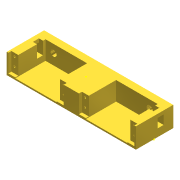
# Autodesk Inventor part: Part4
Saved by Autodesk Inventor 2022 (Build 260153000, 153)
## iProperties
Created: 2021-06-22
Part Number: Part4
Material: Generic
Document SubType Name: Modeling
Designer: Prajwal Patil
Density: 1 g/cm^3
Appearance: Diamond Plate
Author: Prajwal Patil
Autodesk Inventor part; units mm, degrees
ref_plane "YZ Plane" through (0, 0, 0) normal (1, 0, 0) x (0, 1, 0)
ref_plane "XZ Plane" through (0, 0, 0) normal (0, 1, 0) x (-1, 0, 0)
ref_plane "XY Plane" through (0, 0, 0) normal (0, 0, 1) x (1, 0, 0)
sketch "Sketch2" plane through (0, 0, 0) normal (0, 1, 0) x (-1, 0, 0)
  line L0 (77.2994, 22.4824) -> (-85.2606, 22.4824)
  line L1 (-85.2606, 22.4824) -> (-85.2606, -24.5076)
  line L2 (-85.2606, -24.5076) -> (77.2994, -24.5076)
  line L3 (77.2994, -24.5076) -> (77.2994, 22.4824)
  point P0 (0, 0)
  dimension "d0" = 162.56
  dimension "d1" = 46.99
  constraints: 8 end point, 2 parallel, 1 horizontal, 1 perpendicular
  measures "d0" distance of L2.end L1.end
  measures "d1" distance of L1.end L0.end
extrude "Extrusion1" add sketch "Sketch2" along normal blind 25.4
sketch "Sketch3" plane through (0, 25.4, 0) normal (0, 1, 0) x (1, 0, 0)
  point P0 (0, 0)
sketch "Sketch4" plane through (0, 25.4, 0) normal (0, 1, 0) x (1, 0, 0)
  line L0 (85.2606, -22.4824) -> (85.2606, 24.5076) projected
  line L1 (74.5926, -22.4824) -> (74.5926, 15.6176)
  line L2 (74.5926, 15.6176) -> (22.2686, 15.6176)
  line L3 (22.2686, 15.6176) -> (22.2686, -22.4824)
  line L4 (-14.3074, -22.4824) -> (-14.3074, 15.6176)
  line L5 (-14.3074, 15.6176) -> (-66.6314, 15.6176)
  line L6 (-66.6314, 15.6176) -> (-66.6314, -22.4824)
  line L7 (-66.6314, -22.4824) -> (-14.3074, -22.4824)
  line L8 (22.2686, -22.4824) -> (74.5926, -22.4824)
  point P0 (0, 0)
  dimension "d4" = 10.668
  dimension "d5" = 38.1
  dimension "d6" = 52.324
  dimension "d7" = 36.576
  dimension "d8" = 52.324
  constraints: 16 end point, 3 perpendicular, 1 collinear
  measures "d4" distance of L0.start L1.start
  measures "d5" distance of L1.start L1.end
  measures "d6" distance of L1.end L2.end
  measures "d7" distance of L3.end L4.start
  measures "d8" distance of L4.end L5.end
extrude "Extrusion2" cut sketch "Sketch4" against normal blind 23.495
sketch "Sketch5" plane through (0, 25.4, 0) normal (0, 1, 0) x (1, 0, 0)
  line L0 (74.5926, -22.4824) -> (22.2686, -22.4824) projected
  line L1 (22.2686, -22.4824) -> (13.5564, -22.4824)
  line L2 (13.5564, -22.4824) -> (13.5564, -18.6724)
  line L3 (13.5564, -18.6724) -> (22.2686, -18.6724)
  line L4 (22.2686, -18.6724) -> (22.2686, -22.4824)
  line L5 (-14.3074, -22.4824) -> (22.2686, -22.4824) projected
  line L6 (-14.3074, -22.4824) -> (-5.5952, -22.4824)
  line L7 (-5.5952, -22.4824) -> (-5.5952, -18.6724)
  line L8 (-5.5952, -18.6724) -> (-14.3074, -18.6724)
  line L9 (-14.3074, -18.6724) -> (-14.3074, -22.4824)
  line L10 (74.5926, -22.4824) -> (85.2606, -22.4824) projected
  line L11 (74.5926, -22.4824) -> (83.3048, -22.4824)
  line L12 (83.3048, -22.4824) -> (83.3048, -18.6724)
  line L13 (83.3048, -18.6724) -> (74.5926, -18.6724)
  line L14 (74.5926, -18.6724) -> (74.5926, -22.4824)
  line L15 (-66.6314, -22.4824) -> (-66.6314, 15.6176) projected
  line L16 (-66.6314, -22.4824) -> (-75.3436, -22.4824)
  line L17 (-75.3436, -22.4824) -> (-75.3436, -18.6724)
  line L18 (-75.3436, -18.6724) -> (-66.6314, -18.6724)
  line L19 (-66.6314, -18.6724) -> (-66.6314, -22.4824)
  point P0 (0, 0)
  point P1 (-77.2994, -22.4824)
  dimension "d11" = 8.7122
  dimension "d12" = 3.81
  dimension "d13" = 8.7122
  dimension "d14" = 3.81
  dimension "d18" = 8.7122
  dimension "d19" = 8.7122
  dimension "d20" = 3.81
  constraints: 32 end point, 8 parallel, 4 horizontal, 4 perpendicular
  measures "d11" distance of L2.end L3.end
  measures "d12" distance of L1.end L2.end
  measures "d13" distance of L8.end L7.end
  measures "d14" distance of L7.end L6.end
  measures "d18" distance of L13.end L12.end
  measures "d19" distance of L17.end L18.end
  measures "d20" distance of L16.end L17.end
extrude "Extrusion3" cut sketch "Sketch5" against normal blind 22.5552
sketch "Sketch6" plane through (0, 25.4, 0) normal (0, 1, 0) x (1, 0, 0)
  line L0 (74.5926, 12.4426) -> (79.7234, 12.4426)
  line L1 (79.7234, 12.4426) -> (79.7234, 4.8226)
  line L2 (79.7234, 4.8226) -> (74.5926, 4.8226)
  line L3 (74.5926, 12.4426) -> (74.5926, 4.8226)
  line L4 (-66.6314, 12.4426) -> (-71.7622, 12.4426)
  line L5 (-71.7622, 12.4426) -> (-71.7622, 4.8226)
  line L6 (-71.7622, 4.8226) -> (-66.6314, 4.8226)
  line L7 (-66.6314, 4.8226) -> (-66.6314, 12.4426)
  point P0 (0, 0)
  point P1 (74.5926, 15.6176)
  point P2 (-66.6314, 15.6176)
  dimension "d23" = 3.175
  dimension "d24" = 5.1308
  dimension "d25" = 7.62
  dimension "d26" = 3.175
  dimension "d27" = 5.1308
  constraints: 16 end point, 3 perpendicular, 2 horizontal, 1 vertical
  measures "d23" distance of point (74.593, 15.618) L0.start
  measures "d24" distance of L0.start L0.end
  measures "d25" distance of L0.end L1.end
  measures "d26" distance of point (-66.631, 15.618) L4.start
  measures "d27" distance of L4.start L4.end
extrude "Extrusion4" cut sketch "Sketch6" against normal blind 15.875
sketch "Sketch7" plane through (85.2606, 0, 22.4824) normal (1, 0, 0) x (0, 0, -1)
  point P0 (22.4824, 0)
sketch "Sketch8" plane through (85.2606, 0, 22.4824) normal (1, 0, 0) x (0, 0, -1)
  line L0 (27.305, 9.525) -> (34.925, 9.525) projected
  line L1 (27.305, 25.4) -> (27.305, 9.525) projected
  line L2 (34.925, 9.525) -> (27.305, 9.525)
  line L3 (27.305, 9.525) -> (27.305, 20.955)
  line L4 (27.305, 20.955) -> (34.925, 20.955)
  line L5 (38.1, 25.4) -> (38.1, 1.905) projected
  line L6 (34.925, 20.955) -> (34.925, 9.525)
  point P0 (22.4824, 0)
  point P1 (46.99, 0)
  dimension "d32" = 11.43
  constraints: 8 end point, 1 perpendicular, 1 point on line
  measures "d32" distance of L0.start L3.end
extrude "Extrusion5" cut sketch "Sketch8" against normal blind 10.3124
sketch "Sketch10" plane through (-77.2994, 0, -24.5076) normal (-1, 0, 0) x (0, 0, 1)
  line L0 (19.685, 20.955) -> (12.065, 20.955) projected
  line L1 (19.685, 9.525) -> (19.685, 20.955) projected
  line L2 (12.065, 20.955) -> (19.685, 20.955)
  line L3 (19.685, 20.955) -> (19.685, 9.525)
  line L4 (19.685, 9.525) -> (12.065, 9.525)
  line L5 (12.065, 9.525) -> (12.065, 20.955)
  point P0 (24.5076, 0)
  constraints: 8 end point, 2 parallel, 1 horizontal, 1 perpendicular
extrude "Extrusion6" cut sketch "Sketch10" against normal blind 10.3124
sketch "Sketch12" plane through (74.5926, 25.4, 18.6724) normal (0, 0, 1) x (1, 0, 0)
  line L0 (8.7122, -22.5552) -> (4.9022, -22.5552)
  line L1 (-61.0362, 0) -> (-61.0362, -22.5552) projected
  line L2 (-61.0362, -22.5552) -> (-57.2262, -22.5552)
  line L3 (-61.0362, -22.5552) -> (-52.324, -22.5552) projected
  line L4 (8.7122, -22.5552) -> (0, -22.5552) projected
  line L5 (8.7122, -22.5552) -> (4.9022, -22.5552)
  line L6 (10.668, -15.875) -> (0, -15.875) projected
  line L7 (4.9022, -22.5552) -> (12.5222, -22.5552) construction
  circle A0 centre (4.9022, -14.9352) radius 1.27
  circle A1 centre (4.9022, -4.1402) radius 1.27
  circle A2 centre (-57.2262, -4.1402) radius 1.27
  circle A3 centre (-57.2262, -14.9352) radius 1.27
  line L8 (-80.1878, -22.5552) -> (-83.9978, -22.5552)
  line L9 (-80.1878, -22.5552) -> (-88.9, -22.5552) projected
  circle A4 centre (-83.9978, -4.1402) radius 1.27
  circle A5 centre (-83.9978, -14.9352) radius 1.27
  line L10 (-141.224, -22.5552) -> (-149.9362, -22.5552) projected
  line L11 (-149.9362, -22.5552) -> (-146.1262, -22.5552)
  line L12 (-146.1262, -14.9352) -> (-135.3312, -14.9352) construction
  circle A6 centre (-146.1262, -14.9352) radius 1.27
  circle A7 centre (-146.1262, -4.1402) radius 1.27
  point P0 (-74.5926, -25.4)
  dimension "d48" = 3.81
  dimension "d55" = 2.54
  dimension "d56" = 2.54
  dimension "d57" = 3.81
  dimension "d58" = 2.54
  dimension "d59" = 2.54
  dimension "d60" = 3.81
  dimension "d64" = 2.54
  dimension "d65" = 2.54
  constraints: 14 end point, 8 centre point, 3 point on line, 2 horizontal, 1 coincident, 1 collinear
  measures "d48" distance of L1.end L2.end
  measures "d55" diameter of A0
  measures "d56" diameter of A1
  measures "d57" distance of L8.start L8.end
  measures "d58" diameter of A4
  measures "d59" diameter of A5
  measures "d60" distance of L10.end L11.end
  measures "d64" diameter of A6
  measures "d65" diameter of A7
extrude "Extrusion7" cut sketch "Sketch12" against normal blind 10.16
sketch "Sketch13" plane through (22.2686, 25.4, -15.6176) normal (0, 0, 1) x (1, 0, 0)
  line L0 (52.324, -23.495) -> (0, -23.495) projected
  line L1 (52.324, -23.495) -> (42.164, -23.495)
  circle A0 centre (42.164, -10.16) radius 3.81
  line L2 (-88.9, -23.495) -> (-36.576, -23.495) projected
  line L3 (-88.9, -23.495) -> (-78.74, -23.495)
  line L4 (62.992, -25.4) -> (-99.568, -25.4) projected
  line L5 (-88.9, -23.495) -> (-78.74, -23.495) construction
  circle A1 centre (-78.74, -10.16) radius 3.81
  point P0 (-22.2686, -25.4)
  dimension "d68" = 10.16
  dimension "d70" = 7.62
  dimension "d71" = 10.16
  dimension "d72" = 0
  dimension "d73" = 7.62
  constraints: 6 end point, 2 centre point, 1 collinear, 1 horizontal, 1 parallel, 1 point on line
  measures "d68" distance of L0.start L1.end
  measures "d70" diameter of A0
  measures "d71" distance of L2.start L3.end
  measures "d72" distance between parallel lines of L3 L5
  measures "d73" diameter of A1
extrude "Extrusion8" cut sketch "Sketch13" against normal blind 8.89
sketch "Sketch14" plane through (0, 0, 0) normal (0, -1, 0) x (1, 0, 0)
  line L0 (-39.798, -0.8024) -> (112.9368, -0.8024) construction
  line L1 (112.9368, -0.8024) -> (112.9368, -42.123) construction
  line L2 (112.9368, -42.123) -> (-39.798, -42.123) construction
  line L3 (-39.798, -42.123) -> (-39.798, -0.8024) construction
  line L4 (6.2402, -1.1197) -> (5.6265, -1.1197)
  line L5 (5.6265, -1.1197) -> (5.6265, -6.6643)
  line L6 (5.6265, -6.6643) -> (6.2402, -6.6643)
  line L7 (6.2402, -6.6643) -> (6.2402, -3.9544)
  line L8 (6.2402, -3.9544) -> (9.0854, -3.9544)
  line L9 (9.0854, -3.9544) -> (9.0854, -6.6643)
  line L10 (9.0854, -6.6643) -> (9.6992, -6.6643)
  line L11 (9.6992, -6.6643) -> (9.6992, -1.1197)
  line L12 (9.6992, -1.1197) -> (9.0854, -1.1197)
  line L13 (9.0854, -1.1197) -> (9.0854, -3.3719)
  line L14 (9.0854, -3.3719) -> (6.2402, -3.3719)
  line L15 (6.2402, -3.3719) -> (6.2402, -1.1197)
  line L16 (11.582, -3.2158) -> (10.9839, -3.2158)
  line L17 (10.9839, -3.2158) -> (10.9839, -5.2964)
  spline S0 degree 2 poles (10.9839, -5.2964) (10.9787, -5.6084) (11.0983, -6.113) (11.3012, -6.3314) knots 0 0 0 1 2 2 2
  spline S1 degree 2 poles (11.3012, -6.3314) (11.5352, -6.5707) (12.0918, -6.7684) (12.3571, -6.7632) knots 0 0 0 1 2 2 2
  spline S2 degree 2 poles (12.3571, -6.7632) (12.6171, -6.7684) (13.1737, -6.5707) (13.4077, -6.3314) knots 0 0 0 1 2 2 2
  spline S3 degree 2 poles (13.4077, -6.3314) (13.6106, -6.113) (13.7302, -5.6084) (13.725, -5.2964) knots 0 0 0 1 2 2 2
  line L18 (13.725, -5.2964) -> (13.725, -3.2158)
  line L19 (13.725, -3.2158) -> (13.1269, -3.2158)
  line L20 (13.1269, -3.2158) -> (13.1269, -5.2287)
  spline S4 degree 2 poles (13.1269, -5.2287) (13.1321, -5.4108) (13.08, -5.8009) (12.9604, -5.9673) knots 0 0 0 1 2 2 2
  spline S5 degree 2 poles (12.9604, -5.9673) (12.8928, -6.061) (12.6015, -6.2274) (12.3571, -6.2326) knots 0 0 0 1 2 2 2
  spline S6 degree 2 poles (12.3571, -6.2326) (12.1074, -6.2274) (11.8161, -6.061) (11.7485, -5.9673) knots 0 0 0 1 2 2 2
  spline S7 degree 2 poles (11.7485, -5.9673) (11.6289, -5.8009) (11.5768, -5.4108) (11.582, -5.2287) knots 0 0 0 1 2 2 2
  line L21 (11.582, -5.2287) -> (11.582, -3.2158)
  line L22 (14.8589, -6.6643) -> (15.4571, -6.6643)
  line L23 (15.4571, -6.6643) -> (15.4571, -4.7866)
  spline S8 degree 2 poles (15.4571, -4.7866) (15.4519, -4.5682) (15.5507, -4.0532) (15.8784, -3.6735) (16.2113, -3.6631) knots 0 0 0 1 2 3 3 3
  spline S9 degree 2 poles (16.2113, -3.6631) (16.5233, -3.6735) (16.7886, -4.0428) (16.8406, -4.485) (16.8354, -4.6202) knots 0 0 0 1 2 3 3 3
  line L24 (16.8354, -4.6202) -> (16.8354, -6.6643)
  line L25 (16.8354, -6.6643) -> (17.4336, -6.6643)
  line L26 (17.4336, -6.6643) -> (17.4336, -4.745)
  spline S10 degree 2 poles (17.4336, -4.745) (17.4284, -4.5266) (17.5272, -4.0324) (17.8601, -3.6735) (18.1982, -3.6631) knots 0 0 0 1 2 3 3 3
  spline S11 degree 2 poles (18.1982, -3.6631) (18.4739, -3.6683) (18.7391, -3.9544) (18.8171, -4.3653) (18.8119, -4.5682) knots 0 0 0 1 2 3 3 3
  line L27 (18.8119, -4.5682) -> (18.8119, -6.6643)
  line L28 (18.8119, -6.6643) -> (19.4101, -6.6643)
  line L29 (19.4101, -6.6643) -> (19.4101, -4.4798)
  spline S12 degree 2 poles (19.4101, -4.4798) (19.4153, -4.2197) (19.2749, -3.6007) (18.7911, -3.143) (18.2866, -3.1326) knots 0 0 0 1 2 3 3 3
  spline S13 degree 2 poles (18.2866, -3.1326) (18.167, -3.1274) (17.8133, -3.195) (17.418, -3.4291) (17.2515, -3.6891) knots 0 0 0 1 2 3 3 3
  spline S14 degree 2 poles (17.2515, -3.6891) (17.2203, -3.6215) (17.0123, -3.3615) (16.6222, -3.1378) (16.3101, -3.1326) knots 0 0 0 1 2 3 3 3
  spline S15 degree 2 poles (16.3101, -3.1326) (16.0344, -3.1326) (15.6027, -3.3667) (15.4571, -3.5799) knots 0 0 0 1 2 2 2
  line L30 (15.4571, -3.5799) -> (15.4571, -3.2158)
  line L31 (15.4571, -3.2158) -> (14.8589, -3.2158)
  line L32 (14.8589, -3.2158) -> (14.8589, -6.6643)
  spline S16 degree 2 poles (23.1967, -3.7047) (23.1187, -3.5955) (22.817, -3.3302) (22.3489, -3.1378) (22.016, -3.1326) knots 0 0 0 1 2 3 3 3
  spline S17 degree 2 poles (22.016, -3.1326) (21.5687, -3.1326) (20.8093, -3.5383) (20.3411, -4.3393) (20.3359, -4.9375) knots 0 0 0 1 2 3 3 3
  spline S18 degree 2 poles (20.3359, -4.9375) (20.3411, -5.5408) (20.8093, -6.3574) (21.5687, -6.7632) (22.016, -6.7632) knots 0 0 0 1 2 3 3 3
  spline S19 degree 2 poles (22.016, -6.7632) (22.4685, -6.7527) (23.0511, -6.3887) (23.1967, -6.1806) knots 0 0 0 1 2 2 2
  line L33 (23.1967, -6.1806) -> (23.1967, -6.6643)
  line L34 (23.1967, -6.6643) -> (23.7949, -6.6643)
  line L35 (23.7949, -6.6643) -> (23.7949, -3.2158)
  line L36 (23.7949, -3.2158) -> (23.1967, -3.2158)
  line L37 (23.1967, -3.2158) -> (23.1967, -3.7047)
  spline S20 degree 2 poles (22.0836, -3.6631) (22.3541, -3.6631) (22.8794, -3.9336) (23.2227, -4.5006) (23.2279, -4.9427) knots 0 0 0 1 2 3 3 3
  spline S21 degree 2 poles (23.2279, -4.9427) (23.2279, -5.2912) (22.9626, -5.8737) (22.4477, -6.2274) (22.0836, -6.2326) knots 0 0 0 1 2 3 3 3
  spline S22 degree 2 poles (22.0836, -6.2326) (21.5427, -6.2222) (20.9549, -5.5044) (20.9497, -4.9375) knots 0 0 0 1 2 2 2
  spline S23 degree 2 poles (20.9497, -4.9375) (20.9549, -4.5162) (21.267, -3.9492) (21.7819, -3.6631) (22.0836, -3.6631) knots 0 0 0 1 2 3 3 3
  line L38 (24.9288, -6.6643) -> (25.5269, -6.6643)
  line L39 (25.5269, -6.6643) -> (25.5269, -4.8595)
  spline S24 degree 2 poles (25.5269, -4.8595) (25.5217, -4.6618) (25.6049, -4.1417) (25.7766, -3.9284) knots 0 0 0 1 2 2 2
  spline S25 degree 2 poles (25.7766, -3.9284) (25.9066, -3.7776) (26.2239, -3.6579) (26.3799, -3.6631) knots 0 0 0 1 2 2 2
  spline S26 degree 2 poles (26.3799, -3.6631) (26.5776, -3.6631) (26.8585, -3.7984) (26.9469, -3.9128) knots 0 0 0 1 2 2 2
  spline S27 degree 2 poles (26.9469, -3.9128) (27.0457, -4.0532) (27.1081, -4.3861) (27.1029, -4.5422) knots 0 0 0 1 2 2 2
  line L40 (27.1029, -4.5422) -> (27.1029, -6.6643)
  line L41 (27.1029, -6.6643) -> (27.7011, -6.6643)
  line L42 (27.7011, -6.6643) -> (27.7011, -4.5266)
  spline S28 degree 2 poles (27.7011, -4.5266) (27.7063, -4.2405) (27.6283, -3.7932) (27.5034, -3.6059) knots 0 0 0 1 2 2 2
  spline S29 degree 2 poles (27.5034, -3.6059) (27.3422, -3.3719) (26.822, -3.1326) (26.5152, -3.1326) knots 0 0 0 1 2 2 2
  spline S30 degree 2 poles (26.5152, -3.1326) (26.2291, -3.1378) (25.8286, -3.3146) (25.5789, -3.5383) (25.5269, -3.6111) knots 0 0 0 1 2 3 3 3
  line L43 (25.5269, -3.6111) -> (25.5269, -3.2158)
  line L44 (25.5269, -3.2158) -> (24.9288, -3.2158)
  line L45 (24.9288, -3.2158) -> (24.9288, -6.6643)
  line L46 (34.6241, -6.6643) -> (35.3055, -6.6643)
  line L47 (35.3055, -6.6643) -> (32.8192, -0.8544)
  line L48 (32.8192, -0.8544) -> (30.2706, -6.6643)
  line L49 (30.2706, -6.6643) -> (30.9519, -6.6643)
  line L50 (30.9519, -6.6643) -> (31.6177, -5.1039)
  line L51 (31.6177, -5.1039) -> (33.9739, -5.1039)
  line L52 (33.9739, -5.1039) -> (34.6241, -6.6643)
  line L53 (31.857, -4.5214) -> (32.8036, -2.3004)
  line L54 (32.8036, -2.3004) -> (33.7347, -4.5214)
  line L55 (33.7347, -4.5214) -> (31.857, -4.5214)
  line L56 (35.94, -6.6643) -> (36.5382, -6.6643)
  line L57 (36.5382, -6.6643) -> (36.5382, -4.8438)
  spline S31 degree 2 poles (36.5382, -4.8438) (36.5434, -4.4277) (36.6578, -4.0064) (36.7359, -3.9128) knots 0 0 0 1 2 2 2
  spline S32 degree 2 poles (36.7359, -3.9128) (36.8035, -3.8244) (37.0375, -3.6995) (37.2196, -3.6995) knots 0 0 0 1 2 2 2
  spline S33 degree 2 poles (37.2196, -3.6995) (37.2872, -3.6995) (37.4692, -3.7464) (37.5681, -3.814) knots 0 0 0 1 2 2 2
  line L58 (37.5681, -3.814) -> (37.8489, -3.273)
  spline S34 degree 2 poles (37.8489, -3.273) (37.7345, -3.2158) (37.4588, -3.1378) (37.3184, -3.1326) knots 0 0 0 1 2 2 2
  spline S35 degree 2 poles (37.3184, -3.1326) (37.0843, -3.1378) (36.7567, -3.325) (36.5694, -3.5383) (36.5382, -3.5903) knots 0 0 0 1 2 3 3 3
  line L59 (36.5382, -3.5903) -> (36.5382, -3.2158)
  line L60 (36.5382, -3.2158) -> (35.94, -3.2158)
  line L61 (35.94, -3.2158) -> (35.94, -6.6643)
  line L62 (38.4003, -6.6643) -> (38.9984, -6.6643)
  line L63 (38.9984, -6.6643) -> (38.9984, -4.7866)
  spline S36 degree 2 poles (38.9984, -4.7866) (38.9932, -4.5682) (39.0921, -4.0532) (39.4198, -3.6735) (39.7526, -3.6631) knots 0 0 0 1 2 3 3 3
  spline S37 degree 2 poles (39.7526, -3.6631) (40.0647, -3.6735) (40.33, -4.0428) (40.382, -4.485) (40.3768, -4.6202) knots 0 0 0 1 2 3 3 3
  line L64 (40.3768, -4.6202) -> (40.3768, -6.6643)
  line L65 (40.3768, -6.6643) -> (40.975, -6.6643)
  line L66 (40.975, -6.6643) -> (40.975, -4.745)
  spline S38 degree 2 poles (40.975, -4.745) (40.9698, -4.5266) (41.0686, -4.0324) (41.4015, -3.6735) (41.7396, -3.6631) knots 0 0 0 1 2 3 3 3
  spline S39 degree 2 poles (41.7396, -3.6631) (42.0152, -3.6683) (42.2805, -3.9544) (42.3585, -4.3653) (42.3533, -4.5682) knots 0 0 0 1 2 3 3 3
  line L67 (42.3533, -4.5682) -> (42.3533, -6.6643)
  line L68 (42.3533, -6.6643) -> (42.9515, -6.6643)
  line L69 (42.9515, -6.6643) -> (42.9515, -4.4798)
  spline S40 degree 2 poles (42.9515, -4.4798) (42.9567, -4.2197) (42.8162, -3.6007) (42.3325, -3.143) (41.828, -3.1326) knots 0 0 0 1 2 3 3 3
  spline S41 degree 2 poles (41.828, -3.1326) (41.7084, -3.1274) (41.3547, -3.195) (40.9594, -3.4291) (40.7929, -3.6891) knots 0 0 0 1 2 3 3 3
  spline S42 degree 2 poles (40.7929, -3.6891) (40.7617, -3.6215) (40.5537, -3.3615) (40.1636, -3.1378) (39.8515, -3.1326) knots 0 0 0 1 2 3 3 3
  spline S43 degree 2 poles (39.8515, -3.1326) (39.5758, -3.1326) (39.1441, -3.3667) (38.9984, -3.5799) knots 0 0 0 1 2 2 2
  line L70 (38.9984, -3.5799) -> (38.9984, -3.2158)
  line L71 (38.9984, -3.2158) -> (38.4003, -3.2158)
  line L72 (38.4003, -3.2158) -> (38.4003, -6.6643)
  line L73 (46.6184, -6.6643) -> (47.1646, -2.8101)
  line L74 (47.1646, -2.8101) -> (49.0267, -6.8984)
  line L75 (49.0267, -6.8984) -> (50.9148, -2.8101)
  line L76 (50.9148, -2.8101) -> (51.4349, -6.6643)
  line L77 (51.4349, -6.6643) -> (52.0695, -6.6643)
  line L78 (52.0695, -6.6643) -> (51.2061, -0.8076)
  line L79 (51.2061, -0.8076) -> (49.0371, -5.494)
  line L80 (49.0371, -5.494) -> (46.9097, -0.818)
  line L81 (46.9097, -0.818) -> (45.9891, -6.6643)
  line L82 (45.9891, -6.6643) -> (46.6184, -6.6643)
  line L83 (53.2034, -3.2158) -> (53.2034, -6.6643)
  line L84 (53.2034, -6.6643) -> (53.8015, -6.6643)
  line L85 (53.8015, -6.6643) -> (53.8015, -3.2158)
  line L86 (53.8015, -3.2158) -> (53.2034, -3.2158)
  spline S44 degree 2 poles (53.0785, -1.9103) (53.0837, -2.0923) (53.323, -2.3316) (53.4999, -2.3368) knots 0 0 0 1 2 2 2
  spline S45 degree 2 poles (53.4999, -2.3368) (53.6819, -2.3316) (53.9212, -2.0923) (53.9264, -1.9103) knots 0 0 0 1 2 2 2
  spline S46 degree 2 poles (53.9264, -1.9103) (53.9212, -1.7334) (53.6819, -1.4942) (53.4999, -1.489) knots 0 0 0 1 2 2 2
  spline S47 degree 2 poles (53.4999, -1.489) (53.323, -1.4942) (53.0837, -1.7334) (53.0785, -1.9103) knots 0 0 0 1 2 2 2
  line L87 (54.9302, -6.6643) -> (55.5284, -6.6643)
  line L88 (55.5284, -6.6643) -> (55.5284, -4.7866)
  spline S48 degree 2 poles (55.5284, -4.7866) (55.5232, -4.5682) (55.622, -4.0532) (55.9497, -3.6735) (56.2826, -3.6631) knots 0 0 0 1 2 3 3 3
  spline S49 degree 2 poles (56.2826, -3.6631) (56.5947, -3.6735) (56.8599, -4.0428) (56.9119, -4.485) (56.9067, -4.6202) knots 0 0 0 1 2 3 3 3
  line L89 (56.9067, -4.6202) -> (56.9067, -6.6643)
  line L90 (56.9067, -6.6643) -> (57.5049, -6.6643)
  line L91 (57.5049, -6.6643) -> (57.5049, -4.745)
  spline S50 degree 2 poles (57.5049, -4.745) (57.4997, -4.5266) (57.5985, -4.0324) (57.9314, -3.6735) (58.2695, -3.6631) knots 0 0 0 1 2 3 3 3
  spline S51 degree 2 poles (58.2695, -3.6631) (58.5452, -3.6683) (58.8104, -3.9544) (58.8885, -4.3653) (58.8833, -4.5682) knots 0 0 0 1 2 3 3 3
  line L92 (58.8833, -4.5682) -> (58.8833, -6.6643)
  line L93 (58.8833, -6.6643) -> (59.4814, -6.6643)
  line L94 (59.4814, -6.6643) -> (59.4814, -4.4798)
  spline S52 degree 2 poles (59.4814, -4.4798) (59.4866, -4.2197) (59.3462, -3.6007) (58.8625, -3.143) (58.3579, -3.1326) knots 0 0 0 1 2 3 3 3
  spline S53 degree 2 poles (58.3579, -3.1326) (58.2383, -3.1274) (57.8846, -3.195) (57.4893, -3.4291) (57.3229, -3.6891) knots 0 0 0 1 2 3 3 3
  spline S54 degree 2 poles (57.3229, -3.6891) (57.2916, -3.6215) (57.0836, -3.3615) (56.6935, -3.1378) (56.3814, -3.1326) knots 0 0 0 1 2 3 3 3
  spline S55 degree 2 poles (56.3814, -3.1326) (56.1057, -3.1326) (55.674, -3.3667) (55.5284, -3.5799) knots 0 0 0 1 2 2 2
  line L95 (55.5284, -3.5799) -> (55.5284, -3.2158)
  line L96 (55.5284, -3.2158) -> (54.9302, -3.2158)
  line L97 (54.9302, -3.2158) -> (54.9302, -6.6643)
  line L98 (60.6257, -3.2158) -> (60.6257, -6.6643)
  line L99 (60.6257, -6.6643) -> (61.2239, -6.6643)
  line L100 (61.2239, -6.6643) -> (61.2239, -3.2158)
  line L101 (61.2239, -3.2158) -> (60.6257, -3.2158)
  spline S56 degree 2 poles (60.5009, -1.9103) (60.5061, -2.0923) (60.7454, -2.3316) (60.9222, -2.3368) knots 0 0 0 1 2 2 2
  spline S57 degree 2 poles (60.9222, -2.3368) (61.1042, -2.3316) (61.3435, -2.0923) (61.3487, -1.9103) knots 0 0 0 1 2 2 2
  spline S58 degree 2 poles (61.3487, -1.9103) (61.3435, -1.7334) (61.1042, -1.4942) (60.9222, -1.489) knots 0 0 0 1 2 2 2
  spline S59 degree 2 poles (60.9222, -1.489) (60.7454, -1.4942) (60.5061, -1.7334) (60.5009, -1.9103) knots 0 0 0 1 2 2 2
  spline S60 degree 2 poles (65.0469, -3.4655) (64.9221, -3.3667) (64.3863, -3.143) (63.9754, -3.1326) knots 0 0 0 1 2 2 2
  spline S61 degree 2 poles (63.9754, -3.1326) (63.4397, -3.1378) (62.6126, -3.6059) (62.1393, -4.4277) (62.1341, -4.9583) knots 0 0 0 1 2 3 3 3
  spline S62 degree 2 poles (62.1341, -4.9583) (62.1393, -5.4836) (62.6074, -6.295) (63.4345, -6.7579) (63.9754, -6.7632) knots 0 0 0 1 2 3 3 3
  spline S63 degree 2 poles (63.9754, -6.7632) (64.2251, -6.7684) (64.792, -6.6071) (65.0729, -6.4043) knots 0 0 0 1 2 2 2
  line L102 (65.0729, -6.4043) -> (65.0729, -5.6917)
  spline S64 degree 2 poles (65.0729, -5.6917) (64.8284, -5.9777) (64.2355, -6.2326) (63.9598, -6.2326) knots 0 0 0 1 2 2 2
  spline S65 degree 2 poles (63.9598, -6.2326) (63.6477, -6.2326) (63.0964, -5.9413) (62.7531, -5.3744) (62.7479, -4.9531) knots 0 0 0 1 2 3 3 3
  spline S66 degree 2 poles (62.7479, -4.9531) (62.7531, -4.5318) (63.0912, -3.9596) (63.6425, -3.6631) (63.9702, -3.6631) knots 0 0 0 1 2 3 3 3
  spline S67 degree 2 poles (63.9702, -3.6631) (64.2095, -3.6579) (64.8024, -3.8868) (65.0469, -4.1781) knots 0 0 0 1 2 2 2
  line L103 (65.0469, -4.1781) -> (65.0469, -3.4655)
  line L104 (68.0741, -1.1197) -> (68.0741, -6.6643)
  line L105 (68.0741, -6.6643) -> (69.4524, -6.6643)
  spline S68 degree 2 poles (69.4524, -6.6643) (69.7489, -6.6747) (70.4511, -6.5499) (70.7892, -6.3002) knots 0 0 0 1 2 2 2
  spline S69 degree 2 poles (70.7892, -6.3002) (71.0181, -6.1182) (71.3457, -5.5044) (71.3509, -5.1039) knots 0 0 0 1 2 2 2
  spline S70 degree 2 poles (71.3509, -5.1039) (71.3509, -4.8282) (71.1429, -4.2613) (70.68, -3.8088) (70.2951, -3.7099) knots 0 0 0 1 2 3 3 3
  spline S71 degree 2 poles (70.2951, -3.7099) (70.6488, -3.4499) (70.8516, -2.8361) (70.8412, -2.6177) knots 0 0 0 1 2 2 2
  spline S72 degree 2 poles (70.8412, -2.6177) (70.836, -2.2796) (70.6644, -1.8167) (70.4355, -1.5358) (70.3419, -1.4682) knots 0 0 0 1 2 3 3 3
  spline S73 degree 2 poles (70.3419, -1.4682) (70.0246, -1.2341) (69.312, -1.1093) (69.0727, -1.1197) knots 0 0 0 1 2 2 2
  line L106 (69.0727, -1.1197) -> (68.0741, -1.1197)
  line L107 (68.6878, -4.1053) -> (69.3224, -4.1053)
  spline S74 degree 2 poles (69.3224, -4.1053) (69.6501, -4.1053) (70.1078, -4.1833) (70.2587, -4.2717) knots 0 0 0 1 2 2 2
  spline S75 degree 2 poles (70.2587, -4.2717) (70.4355, -4.3549) (70.7268, -4.7554) (70.7372, -5.0831) knots 0 0 0 1 2 2 2
  spline S76 degree 2 poles (70.7372, -5.0831) (70.7372, -5.338) (70.5343, -5.7281) (70.3731, -5.8477) knots 0 0 0 1 2 2 2
  spline S77 degree 2 poles (70.3731, -5.8477) (70.1702, -5.9985) (69.6657, -6.087) (69.3952, -6.0818) knots 0 0 0 1 2 2 2
  line L108 (69.3952, -6.0818) -> (68.6878, -6.0818)
  line L109 (68.6878, -6.0818) -> (68.6878, -4.1053)
  line L110 (68.6878, -1.7022) -> (69.1716, -1.7022)
  spline S78 degree 2 poles (69.1716, -1.7022) (69.2444, -1.697) (69.5825, -1.7386) (69.9622, -1.9103) (70.2378, -2.2952) (70.243, -2.6333) knots 0 0 0 1 2 3 4 4 4
  spline S79 degree 2 poles (70.243, -2.6333) (70.2326, -3.0546) (69.8321, -3.4551) (69.3276, -3.5643) (69.156, -3.5591) knots 0 0 0 1 2 3 3 3
  line L111 (69.156, -3.5591) -> (68.6878, -3.5591)
  line L112 (68.6878, -3.5591) -> (68.6878, -1.7022)
  spline S80 degree 2 poles (73.9464, -6.7632) (74.4718, -6.7579) (75.2936, -6.295) (75.7669, -5.4784) (75.7721, -4.9531) knots 0 0 0 1 2 3 3 3
  spline S81 degree 2 poles (75.7721, -4.9531) (75.7669, -4.4225) (75.2988, -3.6059) (74.477, -3.1378) (73.9464, -3.1326) knots 0 0 0 1 2 3 3 3
  spline S82 degree 2 poles (73.9464, -3.1326) (73.4107, -3.1378) (72.5889, -3.6059) (72.1207, -4.4225) (72.1155, -4.9531) knots 0 0 0 1 2 3 3 3
  spline S83 degree 2 poles (72.1155, -4.9531) (72.1207, -5.4784) (72.5941, -6.295) (73.4159, -6.7579) (73.9464, -6.7632) knots 0 0 0 1 2 3 3 3
  spline S84 degree 2 poles (73.9464, -3.6631) (74.2637, -3.6631) (74.815, -3.9544) (75.1531, -4.5266) (75.1583, -4.9531) knots 0 0 0 1 2 3 3 3
  spline S85 degree 2 poles (75.1583, -4.9531) (75.1531, -5.3744) (74.8098, -5.9413) (74.2585, -6.2326) (73.9464, -6.2326) knots 0 0 0 1 2 3 3 3
  spline S86 degree 2 poles (73.9464, -6.2326) (73.6291, -6.2326) (73.0778, -5.9465) (72.7345, -5.3744) (72.7293, -4.9531) knots 0 0 0 1 2 3 3 3
  spline S87 degree 2 poles (72.7293, -4.9531) (72.7345, -4.5318) (73.0726, -3.9596) (73.6239, -3.6631) (73.9464, -3.6631) knots 0 0 0 1 2 3 3 3
  line L113 (77.8995, -3.762) -> (77.8995, -3.2158)
  line L114 (77.8995, -3.2158) -> (77.3013, -3.2158)
  line L115 (77.3013, -3.2158) -> (77.3013, -1.9675)
  line L116 (77.3013, -1.9675) -> (76.7031, -1.9675)
  line L117 (76.7031, -1.9675) -> (76.7031, -3.2158)
  line L118 (76.7031, -3.2158) -> (76.339, -3.2158)
  line L119 (76.339, -3.2158) -> (76.339, -3.762)
  line L120 (76.339, -3.762) -> (76.7031, -3.762)
  line L121 (76.7031, -3.762) -> (76.7031, -6.6643)
  line L122 (76.7031, -6.6643) -> (77.3013, -6.6643)
  line L123 (77.3013, -6.6643) -> (77.3013, -3.762)
  line L124 (77.3013, -3.762) -> (77.8995, -3.762)
  spline S88 degree 2 poles (23.0094, -18.1983) (23.2019, -18.4531) (23.7949, -18.7756) (24.211, -18.7808) knots 0 0 0 1 2 2 2
  spline S89 degree 2 poles (24.211, -18.7808) (24.7363, -18.7756) (25.4749, -18.2763) (25.865, -17.4597) (25.865, -16.9759) knots 0 0 0 1 2 3 3 3
  spline S90 degree 2 poles (25.865, -16.9759) (25.865, -16.5026) (25.4749, -15.6756) (24.7311, -15.1607) (24.1902, -15.1503) knots 0 0 0 1 2 3 3 3
  spline S91 degree 2 poles (24.1902, -15.1503) (23.9873, -15.1399) (23.3267, -15.3479) (23.0094, -15.712) knots 0 0 0 1 2 2 2
  line L125 (23.0094, -15.712) -> (23.0094, -12.6224)
  line L126 (23.0094, -12.6224) -> (22.4113, -12.6224)
  line L127 (22.4113, -12.6224) -> (22.4113, -18.682)
  line L128 (22.4113, -18.682) -> (23.0094, -18.682)
  line L129 (23.0094, -18.682) -> (23.0094, -18.1983)
  spline S92 degree 2 poles (24.1277, -18.2503) (23.7741, -18.2451) (23.2591, -17.907) (22.9782, -17.3296) (22.9782, -16.9707) knots 0 0 0 1 2 3 3 3
  spline S93 degree 2 poles (22.9782, -16.9707) (22.9834, -16.5546) (23.3163, -15.9773) (23.8365, -15.6808) (24.1225, -15.6808) knots 0 0 0 1 2 3 3 3
  spline S94 degree 2 poles (24.1225, -15.6808) (24.4034, -15.6808) (24.9184, -15.9773) (25.246, -16.5546) (25.2512, -16.9759) knots 0 0 0 1 2 3 3 3
  spline S95 degree 2 poles (25.2512, -16.9759) (25.2512, -17.3296) (24.9808, -17.9018) (24.4814, -18.2451) (24.1277, -18.2503) knots 0 0 0 1 2 3 3 3
  line L130 (26.7752, -20.5909) -> (27.441, -20.5909)
  line L131 (27.441, -20.5909) -> (29.9741, -15.2335)
  line L132 (29.9741, -15.2335) -> (29.3083, -15.2335)
  line L133 (29.3083, -15.2335) -> (28.19, -17.6989)
  line L134 (28.19, -17.6989) -> (26.9677, -15.2335)
  line L135 (26.9677, -15.2335) -> (26.2863, -15.2335)
  line L136 (26.2863, -15.2335) -> (27.8727, -18.3543)
  line L137 (27.8727, -18.3543) -> (26.7752, -20.5909)
  line L138 (35.3991, -13.7199) -> (35.3991, -13.1373)
  line L139 (35.3991, -13.1373) -> (32.091, -13.1373)
  line L140 (32.091, -13.1373) -> (32.091, -13.7199)
  line L141 (32.091, -13.7199) -> (33.4382, -13.7199)
  line L142 (33.4382, -13.7199) -> (33.4382, -18.682)
  line L143 (33.4382, -18.682) -> (34.0519, -18.682)
  line L144 (34.0519, -18.682) -> (34.0519, -13.7199)
  line L145 (34.0519, -13.7199) -> (35.3991, -13.7199)
  spline S96 degree 2 poles (38.6396, -17.5273) (38.5823, -17.6521) (38.4003, -17.9018) (38.2859, -18.0006) knots 0 0 0 1 2 2 2
  spline S97 degree 2 poles (38.2859, -18.0006) (38.135, -18.1255) (37.7865, -18.2503) (37.5785, -18.2503) knots 0 0 0 1 2 2 2
  spline S98 degree 2 poles (37.5785, -18.2503) (37.1156, -18.2451) (36.4966, -17.6209) (36.481, -17.08) knots 0 0 0 1 2 2 2
  line L146 (36.481, -17.08) -> (39.1649, -17.08)
  spline S99 degree 2 poles (39.1649, -17.08) (39.1753, -16.7263) (39.0036, -16.0189) (38.8424, -15.7796) knots 0 0 0 1 2 2 2
  spline S100 degree 2 poles (38.8424, -15.7796) (38.6864, -15.5456) (38.0414, -15.1607) (37.5369, -15.1503) knots 0 0 0 1 2 2 2
  spline S101 degree 2 poles (37.5369, -15.1503) (37.0167, -15.1555) (36.2677, -15.634) (35.8672, -16.4558) (35.8672, -16.9812) knots 0 0 0 1 2 3 3 3
  spline S102 degree 2 poles (35.8672, -16.9812) (35.8776, -17.6157) (36.3718, -18.4115) (37.1468, -18.7808) (37.5681, -18.7808) knots 0 0 0 1 2 3 3 3
  spline S103 degree 2 poles (37.5681, -18.7808) (37.901, -18.7808) (38.4783, -18.5676) (38.7176, -18.3595) knots 0 0 0 1 2 2 2
  spline S104 degree 2 poles (38.7176, -18.3595) (38.8476, -18.2399) (39.0661, -17.9486) (39.1389, -17.803) knots 0 0 0 1 2 2 2
  line L147 (39.1389, -17.803) -> (38.6396, -17.5273)
  spline S105 degree 2 poles (36.5226, -16.5806) (36.6006, -16.1853) (37.1468, -15.686) (37.5369, -15.6808) knots 0 0 0 1 2 2 2
  spline S106 degree 2 poles (37.5369, -15.6808) (37.9218, -15.686) (38.4679, -16.1697) (38.5511, -16.5806) knots 0 0 0 1 2 2 2
  line L148 (38.5511, -16.5806) -> (36.5226, -16.5806)
  spline S107 degree 2 poles (42.7278, -15.7224) (42.6498, -15.6132) (42.3481, -15.3479) (41.88, -15.1555) (41.5471, -15.1503) knots 0 0 0 1 2 3 3 3
  spline S108 degree 2 poles (41.5471, -15.1503) (41.0998, -15.1503) (40.3404, -15.556) (39.8723, -16.357) (39.8671, -16.9551) knots 0 0 0 1 2 3 3 3
  spline S109 degree 2 poles (39.8671, -16.9551) (39.8723, -17.5585) (40.3404, -18.3751) (41.0998, -18.7808) (41.5471, -18.7808) knots 0 0 0 1 2 3 3 3
  spline S110 degree 2 poles (41.5471, -18.7808) (41.9996, -18.7704) (42.5822, -18.4063) (42.7278, -18.1983) knots 0 0 0 1 2 2 2
  line L149 (42.7278, -18.1983) -> (42.7278, -18.682)
  line L150 (42.7278, -18.682) -> (43.326, -18.682)
  line L151 (43.326, -18.682) -> (43.326, -15.2335)
  line L152 (43.326, -15.2335) -> (42.7278, -15.2335)
  line L153 (42.7278, -15.2335) -> (42.7278, -15.7224)
  spline S111 degree 2 poles (41.6147, -15.6808) (41.8852, -15.6808) (42.4105, -15.9513) (42.7538, -16.5182) (42.759, -16.9603) knots 0 0 0 1 2 3 3 3
  spline S112 degree 2 poles (42.759, -16.9603) (42.759, -17.3088) (42.4938, -17.8914) (41.9788, -18.2451) (41.6147, -18.2503) knots 0 0 0 1 2 3 3 3
  spline S113 degree 2 poles (41.6147, -18.2503) (41.0738, -18.2399) (40.486, -17.5221) (40.4808, -16.9551) knots 0 0 0 1 2 2 2
  spline S114 degree 2 poles (40.4808, -16.9551) (40.486, -16.5338) (40.7981, -15.9669) (41.3131, -15.6808) (41.6147, -15.6808) knots 0 0 0 1 2 3 3 3
  line L154 (44.4599, -18.682) -> (45.058, -18.682)
  line L155 (45.058, -18.682) -> (45.058, -16.8043)
  spline S115 degree 2 poles (45.058, -16.8043) (45.0528, -16.5858) (45.1517, -16.0709) (45.4793, -15.6912) (45.8122, -15.6808) knots 0 0 0 1 2 3 3 3
  spline S116 degree 2 poles (45.8122, -15.6808) (46.1243, -15.6912) (46.3896, -16.0605) (46.4416, -16.5026) (46.4364, -16.6379) knots 0 0 0 1 2 3 3 3
  line L156 (46.4364, -16.6379) -> (46.4364, -18.682)
  line L157 (46.4364, -18.682) -> (47.0346, -18.682)
  line L158 (47.0346, -18.682) -> (47.0346, -16.7627)
  spline S117 degree 2 poles (47.0346, -16.7627) (47.0294, -16.5442) (47.1282, -16.0501) (47.4611, -15.6912) (47.7992, -15.6808) knots 0 0 0 1 2 3 3 3
  spline S118 degree 2 poles (47.7992, -15.6808) (48.0748, -15.686) (48.3401, -15.9721) (48.4181, -16.383) (48.4129, -16.5858) knots 0 0 0 1 2 3 3 3
  line L159 (48.4129, -16.5858) -> (48.4129, -18.682)
  line L160 (48.4129, -18.682) -> (49.0111, -18.682)
  line L161 (49.0111, -18.682) -> (49.0111, -16.4974)
  spline S119 degree 2 poles (49.0111, -16.4974) (49.0163, -16.2374) (48.8758, -15.6184) (48.3921, -15.1607) (47.8876, -15.1503) knots 0 0 0 1 2 3 3 3
  spline S120 degree 2 poles (47.8876, -15.1503) (47.7679, -15.1451) (47.4143, -15.2127) (47.019, -15.4467) (46.8525, -15.7068) knots 0 0 0 1 2 3 3 3
  spline S121 degree 2 poles (46.8525, -15.7068) (46.8213, -15.6392) (46.6132, -15.3791) (46.2231, -15.1555) (45.9111, -15.1503) knots 0 0 0 1 2 3 3 3
  spline S122 degree 2 poles (45.9111, -15.1503) (45.6354, -15.1503) (45.2037, -15.3843) (45.058, -15.5976) knots 0 0 0 1 2 2 2
  line L162 (45.058, -15.5976) -> (45.058, -15.2335)
  line L163 (45.058, -15.2335) -> (44.4599, -15.2335)
  line L164 (44.4599, -15.2335) -> (44.4599, -18.682)
  line L165 (53.7339, -18.682) -> (54.3477, -18.682)
  line L166 (54.3477, -18.682) -> (54.3477, -13.1373)
  line L167 (54.3477, -13.1373) -> (53.1254, -13.1373)
  line L168 (53.1254, -13.1373) -> (52.8029, -13.7199)
  line L169 (52.8029, -13.7199) -> (53.7339, -13.7199)
  line L170 (53.7339, -13.7199) -> (53.7339, -18.682)
  line L171 (59.0393, -13.0073) -> (57.1512, -15.6236)
  spline S123 degree 2 poles (57.1512, -15.6236) (56.8495, -16.0657) (56.6831, -16.7367) (56.6935, -16.8979) knots 0 0 0 1 2 2 2
  spline S124 degree 2 poles (56.6935, -16.8979) (56.6935, -17.34) (57.1096, -18.1983) (57.9626, -18.7704) (58.6128, -18.7808) knots 0 0 0 1 2 3 3 3
  spline S125 degree 2 poles (58.6128, -18.7808) (59.1693, -18.7756) (60.0276, -18.2867) (60.5113, -17.4337) (60.5165, -16.8771) knots 0 0 0 1 2 3 3 3
  spline S126 degree 2 poles (60.5165, -16.8771) (60.5113, -16.357) (60.064, -15.5352) (59.2578, -15.0566) (58.722, -15.0514) knots 0 0 0 1 2 3 3 3
  spline S127 degree 2 poles (58.722, -15.0514) (58.592, -15.0514) (58.3475, -15.0879) (58.2331, -15.1295) knots 0 0 0 1 2 2 2
  line L172 (58.2331, -15.1295) -> (59.5022, -13.3558)
  line L173 (59.5022, -13.3558) -> (59.0393, -13.0073)
  spline S128 degree 2 poles (58.6076, -18.2139) (58.2175, -18.2087) (57.6349, -17.8602) (57.3073, -17.2672) (57.3073, -16.8979) knots 0 0 0 1 2 3 3 3
  spline S129 degree 2 poles (57.3073, -16.8979) (57.3177, -16.3414) (58.0198, -15.6288) (58.5972, -15.6184) knots 0 0 0 1 2 2 2
  spline S130 degree 2 poles (58.5972, -15.6184) (59.1745, -15.6288) (59.8923, -16.331) (59.9027, -16.8979) knots 0 0 0 1 2 2 2
  spline S131 degree 2 poles (59.9027, -16.8979) (59.8923, -17.4701) (59.1901, -18.2035) (58.6076, -18.2139) knots 0 0 0 1 2 2 2
  point P0 (0, 0)
  constraints: 2 other
emboss "Emboss1" sketch "Sketch14" operation cut depth 1.016 direction (0, 1, 0)
sketch "Sketch15" plane through (0, 0, 0) normal (0, -1, 0) x (1, 0, 0)
  point P0 (0, 0)
body "Solid1"
